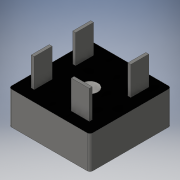
# Autodesk Inventor part: Gleichrichter
Saved by Autodesk Inventor 2016 (Build 200138000, 138)
## iProperties
Created: 2018-05-16
Part Number: Gleichrichter
Material: Generic
Document SubType Name: Modeling
Designer: Phil Erle
Density: 1 g/cm^3
Appearance: Default
Author: Phil Erle
Autodesk Inventor part; units mm, degrees
ref_plane "YZ Plane" through (0, 0, 0) normal (1, 0, 0) x (0, 1, 0)
ref_plane "XZ Plane" through (0, 0, 0) normal (0, 1, 0) x (-1, 0, 0)
ref_plane "XY Plane" through (0, 0, 0) normal (0, 0, 1) x (1, 0, 0)
sketch "Sketch1" plane through (0, 0, 0) normal (0, 0, 1) x (1, 0, 0)
  line L0 (-14.25, -14.25) -> (14.25, -14.25)
  line L1 (14.25, -14.25) -> (14.25, 14.25)
  line L2 (14.25, 14.25) -> (-14.25, 14.25)
  line L3 (-14.25, 14.25) -> (-14.25, -14.25)
  line L4 (-14.25, -14.25) -> (14.25, 14.25) construction
  line L5 (14.25, -14.25) -> (-14.25, 14.25) construction
  point P0 (0, 0)
  dimension "d0" = 28.5
  dimension "d1" = 28.5
  constraints: 12 end point, 2 midpoint, 2 parallel, 1 horizontal, 1 perpendicular
  measures "d0" distance of L2.end L1.end
  measures "d1" distance of L0.end L1.end
extrude "Extrusion1" add sketch "Sketch1" along normal blind 11.5
sketch "Sketch2" plane through (0, 0, 11.5) normal (0, 0, 1) x (1, 0, 0)
  line L0 (-10.15, 4.1) -> (-9.15, 4.1)
  line L1 (-9.15, 4.1) -> (-9.15, 10.4)
  line L2 (-9.15, 10.4) -> (-10.15, 10.4)
  line L3 (-10.15, 10.4) -> (-10.15, 4.1)
  line L4 (-10.15, -10.4) -> (-9.15, -10.4)
  line L5 (-9.15, -10.4) -> (-9.15, -4.1)
  line L6 (-9.15, -4.1) -> (-10.15, -4.1)
  line L7 (-10.15, -4.1) -> (-10.15, -10.4)
  line L8 (3.85, -10.4) -> (10.15, -10.4)
  line L9 (10.15, -10.4) -> (10.15, -9.4)
  line L10 (10.15, -9.4) -> (3.85, -9.4)
  line L11 (3.85, -9.4) -> (3.85, -10.4)
  line L12 (9.15, 10.4) -> (10.15, 10.4)
  line L13 (10.15, 10.4) -> (10.15, 4.1)
  line L14 (10.15, 4.1) -> (9.15, 4.1)
  line L15 (9.15, 4.1) -> (9.15, 10.4)
  line L16 (-9.15, 4.1) -> (-9.15, -4.1) construction
  line L17 (-9.15, 10.4) -> (9.15, 10.4) construction
  point P0 (0, 0)
  point P1 (-9.15, 0)
  point P2 (0, 10.4)
  dimension "d4" = 1
  dimension "d5" = 1
  dimension "d6" = 1
  dimension "d7" = 6.3
  dimension "d8" = 6.3
  dimension "d9" = 6.3
  dimension "d10" = 8.2
  dimension "d11" = 13
  constraints: 36 end point, 8 parallel, 6 point on line, 5 horizontal, 4 perpendicular, 2 midpoint, 1 collinear, 1 horizontal alignment, 1 vertical alignment
  measures "d4" distance of L1.end L2.end
  measures "d5" distance of L12.start L12.end
  measures "d6" distance of L8.end L9.end
  measures "d7" distance of L12.end L13.end
  measures "d8" distance of L6.end L4.start
  measures "d9" distance of L8.start L8.end
  measures "d10" distance between parallel lines of L6 L0
  measures "d11" distance of L8.start L4.end
extrude "Extrusion2" add sketch "Sketch2" along normal blind 10
sketch "Sketch3" plane through (0, 0, 11.5) normal (0, 0, 1) x (1, 0, 0)
  point P0 (0, 0)
  point P1 (0, 0)
  constraints: 1 coincident
hole "Hole1" at (0, 0, 11.5) direction (0, 0, -1) diameter 5.5 depth 8 tip angle 118 clearance for "Countersunk Flat Head Screw DIN EN ISO 2009" size "M5" standard "DIN"
fillet "Fillet1" radius 1 4 edges at (14.25, 14.25, 5.75) (-14.25, 14.25, 5.75) (-14.25, -14.25, 5.75) (14.25, -14.25, 5.75)
body "Solid1"
